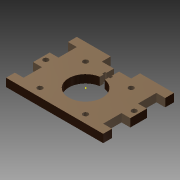
# Autodesk Inventor part: FDM20-BasePrincipal-PortaMotorY-01
Saved by Autodesk Inventor 2015 (Build 190159000, 159)
## iProperties
Created: 2016-02-23
Part Number: FDM20-BasePrincipal-PortaMotorY-01
Material: Generic
Document SubType Name: Modeling
Designer: Proyectil
Density: 1 g/cm^3
Appearance: Brindle
Author: Proyectil
Autodesk Inventor part; units mm, degrees
ref_plane "YZ Plane" through (0, 0, 0) normal (1, 0, 0) x (0, 1, 0)
ref_plane "XZ Plane" through (0, 0, 0) normal (0, 1, 0) x (-1, 0, 0)
ref_plane "XY Plane" through (0, 0, 0) normal (0, 0, 1) x (1, 0, 0)
sketch "Sketch1" plane through (0, 0, 0) normal (0, 0, 1) x (1, 0, 0)
  line L0 (-21.15, 15.9225) -> (-21.15, -15.9225) projected
  line L1 (-20.5642, -17.3367) -> (-17.3367, -20.5642) projected
  line L2 (-15.9225, -21.15) -> (15.9225, -21.15) projected
  line L3 (17.3367, -20.5642) -> (20.5642, -17.3367) projected
  line L4 (21.15, -15.9225) -> (21.15, 15.9225) projected
  line L5 (16.7509, -21.15) -> (21.15, -16.7509)
  line L6 (21.15, -15.9225) -> (21.15, -16.7509)
  line L7 (15.9225, -21.15) -> (16.7509, -21.15)
  line L8 (-17.3367, -20.5642) -> (-16.7509, -21.15)
  line L9 (-15.9225, -21.15) -> (-16.7509, -21.15)
  line L10 (-21.15, -15.9225) -> (-21.15, -16.7509)
  line L11 (-20.5642, -17.3367) -> (-21.15, -16.7509)
  line L12 (15.9225, 21.15) -> (-15.9225, 21.15) projected
  line L13 (21.15, 15.9225) -> (21.15, 21.15)
  line L14 (-21.15, 15.9225) -> (-21.15, 21.15)
  line L15 (-15.9225, 21.15) -> (-21.15, 21.15)
  line L16 (15.9225, 21.15) -> (21.15, 21.15)
  line L17 (21.15, 21.15) -> (-21.15, 21.15)
  line L18 (-21.15, 21.15) -> (-21.15, 27.15)
  line L19 (-21.15, 27.15) -> (21.15, 27.15)
  line L20 (21.15, 27.15) -> (21.15, 21.15)
  circle A0 centre (0, 0) radius 11.5
  circle A1 centre (-15.5563, 15.5563) radius 1.75
  line L21 (-15.5563, 15.5563) -> (0, 0) construction
  circle A2 centre (-15.5563, -15.5563) radius 1.75
  circle A3 centre (15.5563, -15.5563) radius 1.75
  circle A4 centre (15.5563, 15.5563) radius 1.75
  dimension "d0" = 6
  dimension "d1" = 23
  dimension "d2" = 3.5
  dimension "d3" = 45
  dimension "d4" = 22
  dimension "d7" = 360
  constraints: 32 end point, 11 collinear, 5 centre point, 2 horizontal, 2 parallel, 1 coincident, 1 perpendicular, 9 other
  measures "d0" distance of L17.end L18.end
  measures "d1" diameter of A0
  measures "d2" diameter of A1
  measures "d3" angle of L12 L21
  measures "d4" distance of L21.start L21.end
extrude "Extrusion1" add sketch "Sketch1" along normal blind 5.5
sketch "Sketch2" plane through (0, 0, 5.5) normal (0, 0, 1) x (1, 0, 0)
  line L0 (21.15, 27.15) -> (-21.15, 27.15) projected
  line L1 (-10, 27.15) -> (10, 27.15)
  line L2 (10, 27.15) -> (10, 21.0704)
  line L3 (10, 21.0704) -> (-10, 21.0704)
  line L4 (-10, 21.0704) -> (-10, 27.15)
  line L5 (0, 27.15) -> (0, 0) construction
  dimension "d11" = 20
  dimension "d12" = 10
  constraints: 10 end point, 2 parallel, 2 perpendicular, 1 horizontal, 1 midpoint, 1 point on line
  measures "d11" distance of L2.end L3.end
  measures "d12" distance between parallel lines of L5 L4
extrude "Extrusion2" cut sketch "Sketch2" against normal up to next
sketch "Sketch3" plane through (0, 0, 5.5) normal (0, 0, 1) x (1, 0, 0)
  line L0 (-21.15, -16.7509) -> (-16.7509, -21.15) projected
  line L1 (-21.15, 27.15) -> (-21.15, -16.7509) projected
  line L2 (21.15, -16.7509) -> (21.15, 27.15) projected
  line L3 (16.7509, -21.15) -> (21.15, -16.7509) projected
  line L4 (-16.7509, -21.15) -> (-33.15, -21.15)
  line L5 (-33.15, -21.15) -> (-33.15, 27.15)
  line L6 (-33.15, 27.15) -> (-21.15, 27.15)
  line L7 (21.15, 27.15) -> (33.15, 27.15)
  line L8 (33.15, 27.15) -> (33.15, -21.15)
  line L9 (33.15, -21.15) -> (16.7509, -21.15)
  point P0 (0, 0)
  dimension "d15" = 12
  dimension "d16" = 12
  constraints: 12 end point, 4 perpendicular, 2 point on line, 1 horizontal
  measures "d15" distance of L5.end L1.start
  measures "d16" distance of L2.end L7.end
extrude "Extrusion3" add sketch "Sketch3" against normal up to surface (5.5 mm away)
sketch "Sketch4" plane through (0, 0, 5.5) normal (0, 0, 1) x (1, 0, 0)
  line L0 (-33.15, -21.15) -> (-33.15, 27.15) projected
  line L1 (-33.15, -15.15) -> (-27.15, -15.15)
  line L2 (-27.15, -15.15) -> (-27.15, -2.65)
  line L3 (-27.15, -2.65) -> (-33.15, -2.65)
  line L4 (-33.15, -2.65) -> (-33.15, -15.15)
  line L5 (33.15, -21.15) -> (-33.15, -21.15) projected
  line L6 (-33.15, 21.15) -> (-27.15, 21.15)
  line L7 (-27.15, 21.15) -> (-27.15, 8.65)
  line L8 (-27.15, 8.65) -> (-33.15, 8.65)
  line L9 (-33.15, 8.65) -> (-33.15, 21.15)
  line L10 (33.15, 27.15) -> (33.15, -21.15) projected
  line L11 (33.15, -15.15) -> (27.15, -15.15)
  line L12 (27.15, -15.15) -> (27.15, -2.65)
  line L13 (27.15, -2.65) -> (33.15, -2.65)
  line L14 (33.15, -2.65) -> (33.15, -15.15)
  line L15 (33.15, 8.65) -> (27.15, 8.65)
  line L16 (27.15, 8.65) -> (27.15, 21.15)
  line L17 (27.15, 21.15) -> (33.15, 21.15)
  line L18 (33.15, 21.15) -> (33.15, 8.65)
  line L19 (-10, 27.15) -> (-33.15, 27.15) projected
  point P0 (0, 0)
  dimension "d19" = 6
  dimension "d20" = 12.5
  dimension "d21" = 6
  dimension "d22" = 12.5
  dimension "d23" = 6
  dimension "d24" = 6
  constraints: 32 end point, 8 parallel, 5 collinear, 5 point on line, 4 horizontal, 4 perpendicular
  measures "d19" distance of L3.end L2.end
  measures "d20" distance of L2.end L1.end
  measures "d21" distance between parallel lines of L5 L1
  measures "d22" distance of L6.end L7.end
  measures "d23" distance between parallel lines of L19 L6
  measures "d24" distance of L16.end L17.end
extrude "Extrusion4" cut sketch "Sketch4" against normal up to surface (5.5 mm away)
sketch "Sketch5" plane through (0, 0, 5.5) normal (0, 0, 1) x (1, 0, 0)
  line L0 (-27.15, -2.65) -> (-33.15, -2.65) construction
  line L1 (-30.15, -2.65) -> (-30.15, 8.65) construction
  line L2 (-33.15, 8.65) -> (-27.15, 8.65) construction
  line L3 (27.15, -2.65) -> (33.15, -2.65) construction
  line L4 (30.15, -2.65) -> (30.15, 8.65) construction
  line L5 (27.15, 8.65) -> (33.15, 8.65) construction
  circle A0 centre (30.15, 3) radius 1.75
  circle A1 centre (-30.15, 3) radius 1.75
  point P0 (0, 0)
  dimension "d27" = 3.5
  dimension "d28" = 3.5
  constraints: 6 midpoint, 4 end point, 2 centre point
  measures "d27" diameter of A0
  measures "d28" diameter of A1
extrude "Extrusion5" cut sketch "Sketch5" against normal up to next
sketch "Sketch6" plane through (0, 0, 5.5) normal (0, 0, 1) x (1, 0, 0)
  point P0 (0, 0)
sketch "Sketch7" plane through (0, 0, 5.5) normal (0, 0, 1) x (1, 0, 0)
  line L0 (10, 21.0704) -> (-10, 21.0704) construction
  line L1 (0, 21.0704) -> (0, 11.5638) construction
  line L2 (-1.75, 21.0704) -> (-1.75, 16.0704)
  line L3 (-1.75, 16.0704) -> (-2.75, 16.0704)
  line L4 (-2.75, 16.0704) -> (-2.75, 14.0704)
  line L5 (-2.75, 14.0704) -> (-1.75, 14.0704)
  line L6 (-1.75, 14.0704) -> (-1.75, 11.3661)
  circle A0 centre (0, 0) radius 11.5 construction
  line L7 (1.75, 21.0704) -> (1.75, 16.0704)
  line L8 (1.75, 16.0704) -> (2.75, 16.0704)
  line L9 (2.75, 16.0704) -> (2.75, 14.0704)
  line L10 (2.75, 14.0704) -> (1.75, 14.0704)
  line L11 (1.75, 14.0704) -> (1.75, 11.3661)
  arc A1 (1.75, 11.3661) -> (-1.75, 11.3661) centre (0, 0) ccw
  line L12 (-1.75, 21.0704) -> (1.75, 21.0704)
  dimension "d31" = 5
  dimension "d32" = 2
  dimension "d33" = 3.5
  dimension "d34" = 1.75
  dimension "d35" = 5.5
  dimension "d36" = 2.75
  constraints: 24 end point, 7 perpendicular, 6 point on line, 4 point on circle, 3 collinear, 2 vertical, 1 centre point, 1 coincident, 1 midpoint
  measures "d31" distance of L2.start L2.end
  measures "d32" distance of L3.end L4.end
  measures "d33" distance between parallel lines of L7 L2
  measures "d34" distance between parallel lines of L1 L2
  measures "d35" distance between parallel lines of L9 L4
  measures "d36" distance between parallel lines of L1 L4
extrude "Extrusion6" cut sketch "Sketch7" against normal up to next
equation "\"d12\" = 0.5 * d11"
equation "\"d34\" = 0.5 * d33"
equation "\"d36\" = 0.5 * d35"
body "Solid1"
